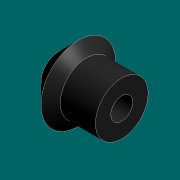
# Autodesk Inventor part: P07
Saved by Autodesk Inventor 2012 SP1 (Build 160190100, 190)
## iProperties
Created: 2011-05-10
Part Number: P07
Material: Acetal Resin, White
Document SubType Name: Modeling
Designer: sta
Density: 1.42 g/cm^3
Description: Kegelrad
Mass: 2.15127 g
Surface Area: 10.4483 cm^2
Volume: 1.51498 cm^3
Title: Kart
Author: sta
Autodesk Inventor part; units mm, degrees
ref_plane "YZ Plane" through (0, 0, 0) normal (1, 0, 0) x (0, 1, 0)
ref_plane "XZ Plane" through (0, 0, 0) normal (0, 1, 0) x (-1, 0, 0)
sketch "Sketch1" plane through (0, 0, 0) normal (0, 0, 1) x (1, 0, 0)
  line L0 (0, 4) -> (4.5, 8.5)
  line L1 (4.5, 8.5) -> (6.4, 6)
  line L2 (6.4, 6) -> (14.4, 6)
  line L3 (14.4, 6) -> (14.4, 0)
  line L4 (14.4, 0) -> (0, 0)
  line L5 (-2.988, 0) -> (27.6356, 0) construction
  line L6 (0, 4) -> (0, 0)
  line L7 (0, 2.5) -> (14.4, 2.5)
  dimension "d0" = 17
  dimension "d1" = 45
  dimension "d2" = 90
  dimension "d3" = 8
  dimension "d5" = 12
  dimension "d6" = 14.4
  dimension "d7" = 5
  dimension "d9" = 8
  constraints: 16 end point, 3 point on line, 2 parallel, 1 coincident, 1 collinear, 1 horizontal
  measures "d0" diameter of L0.end L5
  measures "d1" angle of L6 L0
  measures "d2" angle of L4 L6
  measures "d3" diameter of L0.start L5
  measures "d5" diameter of L2 L5
  measures "d6" distance between parallel lines of L3 L6
  measures "d7" diameter of L7 L5
  measures "d9" distance from line of L1.end L3
revolve "Revolution1" add sketch "Sketch1" angle 360 about axis through (-2.988, 0, 0) along (1, 0, 0) contours L0 L1 L2 L3 L7 L6
ref_plane "Work Plane1" through (10.4, 0, 6) normal (0, 0, 1) x (1, 0, 0)
sketch "Sketch3" plane through (10.4, 0, 6) normal (0, 0, 1) x (1, 0, 0)
  line L0 (4, -6) -> (4, 6) construction
  line L1 (5.4316, 0) -> (-5.4316, 0)
  point P0 (-10.4, 0)
  point P1 (0, 0)
  dimension "d12" = 4
  constraints: 2 end point, 1 midpoint, 1 perpendicular
  measures "d12" distance from line of L0 point (0, 0)
hole "Hole1" at (10.4, 0, 6) direction (0, 0, -1) diameter 2 end through all
body "Solid1"
